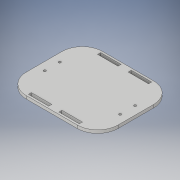
# Autodesk Inventor part: base_plate
Saved by Autodesk Inventor 2017 (Build 210142000, 142)
## iProperties
Created: 2017-06-15
Part Number: base_plate
Material: Generic
Document SubType Name: Modeling
Designer: millerid
Density: 1 g/cm^3
Appearance: Default
Author: millerid
Autodesk Inventor part; units mm, degrees
ref_plane "YZ Plane" through (0, 0, 0) normal (1, 0, 0) x (0, 1, 0)
ref_plane "XZ Plane" through (0, 0, 0) normal (0, 1, 0) x (-1, 0, 0)
ref_plane "XY Plane" through (0, 0, 0) normal (0, 0, 1) x (1, 0, 0)
sketch "Sketch1" plane through (0, 0, 0) normal (0, 1, 0) x (-1, 0, 0)
  line L0 (20, 0) -> (70, 0)
  line L1 (90, -20) -> (90, -55)
  line L2 (70, -75) -> (20, -75)
  line L3 (0, -55) -> (0, -20)
  line L4 (70, -70) -> (50, -70)
  line L5 (50, -70) -> (50, -73)
  line L6 (50, -73) -> (70, -73)
  line L7 (70, -73) -> (70, -70)
  line L8 (70, -2) -> (50, -2)
  line L9 (50, -2) -> (50, -5)
  line L10 (50, -5) -> (70, -5)
  line L11 (70, -5) -> (70, -2)
  circle A0 centre (82, -30.134) radius 1.143
  circle A1 centre (82, -44.866) radius 1.143
  circle A2 centre (8, -30.134) radius 1.143
  circle A3 centre (8, -44.866) radius 1.143
  arc A4 (90, -20) -> (70, 0) centre (70, -20) ccw
  arc A5 (0, -55) -> (20, -75) centre (20, -55) ccw
  arc A6 (70, -75) -> (90, -55) centre (70, -55) ccw
  arc A7 (20, 0) -> (0, -20) centre (20, -20) ccw
  line L12 (40, -2) -> (20, -2)
  line L13 (20, -2) -> (20, -5)
  line L14 (20, -5) -> (40, -5)
  line L15 (40, -5) -> (40, -2)
  line L16 (40, -70) -> (20, -70)
  line L17 (20, -70) -> (20, -73)
  line L18 (20, -73) -> (40, -73)
  line L19 (40, -73) -> (40, -70)
  point P0 (0, 0)
  point P1 (90, -75)
  point P2 (90, 0)
  point P3 (0, -75)
  dimension "d0" = 90
  dimension "d1" = 75
  dimension "d2" = 20
  dimension "d3" = 3
  dimension "d4" = 20
  dimension "d5" = 3
  dimension "d6" = 2
  dimension "d7" = 2
  dimension "d8" = 20
  dimension "d9" = 2.286
  dimension "d10" = 2.286
  dimension "d11" = 14.732
  dimension "d12" = 30.134
  dimension "d13" = 8
  dimension "d14" = 8
  dimension "d15" = 2.286
  dimension "d16" = 2.286
  dimension "d17" = 8
  dimension "d18" = 8
  dimension "d19" = 20
  dimension "d20" = 20
  dimension "d21" = 20
  dimension "d24" = 20
  dimension "d25" = 20
  constraints: 40 end point, 10 parallel, 8 centre point, 8 point on circle, 8 point on line, 8 tangent, 7 collinear, 5 horizontal, 5 perpendicular, 1 equal radius
  measures "d0" distance of point (90, -75) point (0, -75)
  measures "d1" distance of point (90, 0) point (90, -75)
  measures "d2" distance of L6.end L5.end
  measures "d3" distance of L5.end L4.end
  measures "d4" distance of L10.end L9.end
  measures "d5" distance of L9.end L8.end
  measures "d6" distance between parallel lines of L0 L8
  measures "d7" distance between parallel lines of L2 L6
  measures "d8" distance between parallel lines of L11 L1
  measures "d9" diameter of A0
  measures "d10" diameter of A1
  measures "d11" distance of A1.centre A0.centre
  measures "d12" distance from line of L0 A0.centre
  measures "d13" distance from line of L1 A1.centre
  measures "d14" distance from line of A0.centre L1
  measures "d15" diameter of A2
  measures "d16" diameter of A3
  measures "d17" distance from line of L3 A2.centre
  measures "d18" distance from line of L3 A3.centre
  measures "d19" radius of A4
  measures "d20" radius of A5
  measures "d21" radius of A7
  measures "d24" distance of L14.end L13.end
  measures "d25" distance between parallel lines of L13 L3
extrude "Extrusion2" add sketch "Sketch1" along normal blind 3
equation "\"d10\" = d9"
equation "\"d12\" = -0.5 * d11 + 0.5 * d1"
equation "\"d15\" = d9"
equation "\"d16\" = d9"
body "Solid2"
